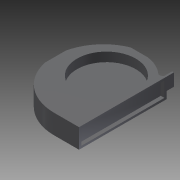
# Autodesk Inventor part: Ventilador
Saved by Autodesk Inventor 2014 (Build 180170000, 170)
## iProperties
Created: 2016-06-30
Part Number: Ventilador
Material: Generic
Document SubType Name: Modeling
Designer: Rubén
Density: 1 g/cm^3
Appearance: Smooth - Medium Gray
Author: Rubén
Autodesk Inventor part; units mm, degrees
ref_plane "YZ Plane" through (0, 0, 0) normal (1, 0, 0) x (0, 1, 0)
ref_plane "XZ Plane" through (0, 0, 0) normal (0, 1, 0) x (-1, 0, 0)
ref_plane "XY Plane" through (0, 0, 0) normal (0, 0, 1) x (1, 0, 0)
sketch "Sketch1" plane through (0, 0, 0) normal (0, 1, 0) x (-1, 0, 0)
  line L0 (0, 0) -> (40, 0)
  line L1 (40, 0) -> (40, 52)
  line L2 (40, 52) -> (0, 52)
  line L3 (0, 52) -> (0, 0)
  dimension "d0" = 40
  dimension "d1" = 52
  constraints: 8 end point, 2 parallel, 1 horizontal, 1 perpendicular
  measures "d0" distance of L2.end L1.end
  measures "d1" distance of L1.end L0.end
extrude "Extrusion1" add sketch "Sketch1" along normal blind 10.7
sketch "Sketch2" plane through (0, 10.7, 0) normal (0, 1, 0) x (1, 0, 0)
  line L0 (0, 0) -> (-40, 0) projected
  line L1 (-40, 0) -> (-40, -52) projected
  line L2 (-40, -52) -> (0, -52) projected
  line L3 (0, -52) -> (0, 0) projected
  arc A0 (-23.7, 0) -> (-40, -19.4) centre (-13.6141, -25.0219) ccw
  line L4 (-40, -19.4) -> (0, -19.4) construction
  arc A1 (-40, -30.6438) -> (-13.6141, -52) centre (-13.6141, -25.0219) ccw
  arc A2 (-40, -19.4) -> (-40, -30.6438) centre (-13.6141, -25.0219) ccw
  arc A3 (0, -9.1718) -> (-14.5, 0) centre (-17, -20) ccw
  line L5 (0, -4) -> (-2.8506, -5.6458)
  dimension "d8" = 16.3
  dimension "d9" = 19.4
  dimension "d12" = 20
  dimension "d13" = 17
  dimension "d14" = 14.5
  dimension "d15" = 4
  dimension "d16" = 30
  constraints: 10 point on circle, 8 point on line, 4 centre point, 4 end point, 2 tangent, 1 perpendicular
  measures "d8" distance from line of L1 A0.start
  measures "d9" distance between parallel lines of L4 L0
  measures "d12" distance from line of L0 A3.centre
  measures "d13" distance from line of L3 A3.centre
  measures "d14" distance from line of L3 A3.end
  measures "d15" distance from line of L5.start L0
  measures "d16" angle of L0 L5
extrude "Extrusion2" cut sketch "Sketch2" against normal through all contours L3 L5 A3 L0 | A0 L1 L0 | A1 L2 L1
sketch "Sketch4" plane through (0, 10.7, 0) normal (0, 1, 0) x (1, 0, 0)
  line L0 (0, -52) -> (0, -4) projected
  arc A0 (-2.8506, -5.6458) -> (-14.5, 0) centre (-17, -20) ccw projected
  line L1 (-14.5, 0) -> (-23.7, 0) projected
  circle A1 centre (-17, -20) radius 16.1
  line L2 (-3, -12.0495) -> (-3, -27.9505)
  point P0 (0, 0)
  dimension "d17" = 32.2
  dimension "d18" = 3
  constraints: 2 end point, 2 point on circle, 1 centre point, 1 coincident, 1 perpendicular
  measures "d17" diameter of A1
  measures "d18" distance between parallel lines of L0 L2
extrude "Extrusion3" cut sketch "Sketch4" against normal blind 5 contours L2 A1 picked at (-14.3987, -21.2686)
sketch "Sketch5" plane through (0, 0, 52) normal (1, 0, 0) x (0, 0, -1)
  line L0 (48, 0) -> (48, 10.7) projected
  line L1 (0, 10.7) -> (48, 10.7) projected
  line L2 (0, 0) -> (0, 10.7) projected
  line L3 (0, 0) -> (48, 0) projected
  line L4 (46.8, 9.5) -> (46.8, 1.2)
  line L5 (46.8, 1.2) -> (1.2, 1.2)
  line L6 (1.2, 1.2) -> (1.2, 9.5)
  line L7 (1.2, 9.5) -> (46.8, 9.5)
  point P0 (52, 0)
  dimension "d21" = 1.2
  constraints: 8 end point, 3 other
  measures "d21" distance between parallel lines of L1 L7
extrude "Extrusion4" cut sketch "Sketch5" against normal blind 2 contours L4 L5 L6 L7
sketch "Sketch6" plane through (-14.5, 0, 0) normal (0, 0, -1) x (-1, 0, 0)
  line L0 (0, 10.7) -> (9.2, 10.7) projected
  line L1 (-11.6494, 0) -> (-14.5, 0) projected
  line L2 (-11.6494, 10.7) -> (-11.6494, 0) projected
  line L3 (-14.5, 10.7) -> (-11.6494, 10.7) projected
  line L4 (-14.5, 0) -> (-14.5, 10.7) projected
  line L5 (0, 0) -> (-11.6494, 0) projected
  line L6 (0, 10.7) -> (0, 0) projected
  line L7 (-11.6494, 10.7) -> (0, 10.7) projected
  line L8 (-11.6494, 10.7) -> (-11.6494, 0) projected
  line L9 (0, 3.9) -> (-14.5, 3.9)
  line L10 (0, 5.5) -> (-13.5, 5.5)
  line L11 (-13.5, 5.5) -> (-13.5, 10.7)
  dimension "d24" = 1
  dimension "d25" = 1.6
  dimension "d26" = 3.9
  constraints: 6 end point, 4 point on line, 3 perpendicular, 1 parallel
  measures "d24" distance between parallel lines of L4 L11
  measures "d25" distance between parallel lines of L9 L10
  measures "d26" distance between parallel lines of L5 L9
extrude "Extrusion5" add sketch "Sketch6" against normal up to next contours L9 L4 L3 L11 L10 L2 | L2 L10 L6 L9
sketch "Sketch7" plane through (-14.5, 5.5, 0) normal (0, 1, 0) x (1, 0, 0)
  line L0 (0, 0) -> (13.5, 0) projected
  circle A0 centre (11, -2) radius 1.45
  line L1 (14.5, 0) -> (14.5, -4) projected
  dimension "d29" = 2.9
  dimension "d30" = 3.5
  dimension "d31" = 2
  constraints: 1 centre point
  measures "d29" diameter of A0
  measures "d30" distance from line of L1 A0.centre
  measures "d31" distance from line of L0 A0.centre
extrude "Extrusion6" cut sketch "Sketch7" against normal through all
body "Solid1"
